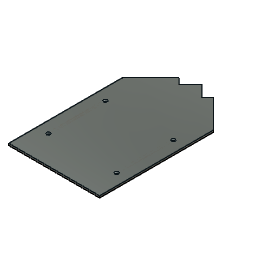
PCB (v2) (Autodesk Fusion 360 design; units mm, degrees)
Autodesk Fusion 360 part; units mm, degrees
sketch "Sketch1" plane through (0, 0, 0) normal (0, 0, 1) x (1, 0, 0)
  line L0 (0, 0) -> (80, 0)
  line L1 (80, 0) -> (80, 100)
  line L2 (80, 100) -> (0, 100)
  line L3 (0, 100) -> (0, 0)
  line L4 (40, 100) -> (40, 130)
  line L5 (40, 130) -> (50, 120)
  line L6 (50, 120) -> (55, 125)
  line L7 (55, 125) -> (65, 115)
  line L8 (65, 115) -> (80, 100)
  line L9 (40, 130) -> (30, 120)
  line L10 (30, 120) -> (25, 125)
  line L11 (25, 125) -> (0, 100)
  constraint horizontal L0
  constraint vertical L1
  constraint horizontal L2
  constraint vertical L3
  constraint coincident L0.start L3.end
  constraint midpoint L2 L4.start
  constraint perpendicular L2 L4
  constraint perpendicular L5 L6
  constraint perpendicular L6 L7
  constraint parallel L7 L8
  constraint perpendicular L5 L9
  constraint perpendicular L9 L10
  constraint perpendicular L10 L11
extrude "Extrude1" add sketch "Sketch1" along normal blind 6
extrude "Extrude2" cut 1 faces at (26.6667, 66.6667, 6) along direction (0, 0, -1) blind 4.4
sketch "Sketch2" plane through (0, 0, 1.6) normal (0, 0, 1) x (-1, 0, 0)
  line L0 (-40, -130) -> (-30, -120)
  line L1 (-30, -120) -> (-25, -125)
  line L2 (-25, -125) -> (0, -100)
  line L3 (0, -100) -> (0, 0)
  line L4 (0, 0) -> (-80, 0)
  line L5 (-80, 0) -> (-80, -100)
  line L6 (-80, -100) -> (-55, -125)
  line L7 (-55, -125) -> (-50, -120)
  line L8 (-50, -120) -> (-40, -130)
  line L9 (-80, -100) -> (0, 0) construction
  line L10 (0, -100) -> (-80, 0) construction
  line L11 (-70, -75) -> (-10, -75) construction
  line L12 (-10, -75) -> (-10, -25) construction
  line L13 (-10, -25) -> (-70, -25) construction
  line L14 (-70, -25) -> (-70, -75) construction
  line L15 (-70, -75) -> (-10, -25) construction
  line L16 (-10, -75) -> (-70, -25) construction
  circle A0 centre (-10, -75) radius 1.65
  circle A1 centre (-70, -75) radius 1.65
  circle A2 centre (-10, -25) radius 1.65
  circle A3 centre (-70, -25) radius 1.65
  point P0 (-40, -50)
  dimension "d5" = 60
  dimension "d6" = 50
  dimension "d7" = 3.3
  dimension "d8" = 3.3
  dimension "d9" = 3.3
  dimension "d10" = 3.3
  constraint coincident L5.end L6.start
  constraint coincident L3.end L4.start
  constraint coincident L2.end L3.start
  constraint coincident L4.end L5.start
  constraint horizontal L11
  constraint perpendicular L11 L12
  constraint parallel L11 L13
  constraint parallel L12 L14
  constraint coincident L15 P0
  constraint coincident L16 P0
  constraint midpoint L10 P0
  constraint coincident L11.end L12.start
  constraint coincident L11.start L14.end
  constraint coincident L12.end L13.start
  constraint coincident L13.end L14.start
  measures "d5" distance of L11.start L11.end
  measures "d6" distance of L11.start L13.end
  measures "d7" diameter of A0
  measures "d8" diameter of A1
  measures "d9" diameter of A2
  measures "d10" diameter of A3
extrude "Extrude3" cut sketch "Sketch2" against normal blind 55 contours A0 | A1 | A2 | A3
sketch "Sketch3" plane through (0, 0, 1.6) normal (0, 0, 1) x (-1, 0, 0)
  circle A0 centre (-10, -25) radius 1.65
  circle A1 centre (-10, -75) radius 1.65
  circle A2 centre (-70, -25) radius 1.65
  circle A3 centre (-70, -75) radius 1.65
  line L0 (-40, -130) -> (-30, -120)
  line L1 (-30, -120) -> (-25, -125)
  line L2 (-25, -125) -> (0, -100)
  line L3 (0, -100) -> (0, 0)
  line L4 (0, 0) -> (-80, 0)
  line L5 (-80, 0) -> (-80, -100)
  line L6 (-80, -100) -> (-55, -125)
  line L7 (-55, -125) -> (-50, -120)
  line L8 (-50, -120) -> (-40, -130)
sketch "Sketch4" plane through (0, 0, 1.6) normal (0, 0, 1) x (1, 0, 0)
